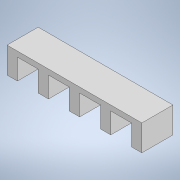
# Autodesk Inventor part: chamber
Saved by Autodesk Inventor 2021 (Build 250183000, 183)
## iProperties
Created: 2022-01-02
Part Number: chamber
Material: 一般
Document SubType Name: Modeling
Designer: shibu
Density: 1 g/cm^3
Appearance: 既定
Author: shibu
Autodesk Inventor part; units mm, degrees
ref_plane "YZ Plane" through (0, 0, 0) normal (1, 0, 0) x (0, 1, 0)
ref_plane "XZ Plane" through (0, 0, 0) normal (0, 1, 0) x (-1, 0, 0)
ref_plane "XY Plane" through (0, 0, 0) normal (0, 0, 1) x (1, 0, 0)
sketch "スケッチ1" plane through (0, 0, 0) normal (0, 0, 1) x (1, 0, 0)
  line L0 (0, 0) -> (-15, 0)
  line L1 (-15, 0) -> (-15, 20)
  line L2 (-15, 20) -> (0, 20)
  line L3 (0, 20) -> (0, 0)
  line L4 (0, 0) -> (0, 43.6966) construction
  line L5 (-15, 12.5) -> (-20, 12.5)
  line L6 (-20, 12.5) -> (-20, 0)
  line L7 (-30, 0) -> (-30, 12.5)
  line L8 (-30, 0) -> (-20, 0)
  line L9 (23.8812, 0) -> (-169.724, 0) construction
  line L10 (-45, 0) -> (-45, 12.5)
  line L11 (-45, 0) -> (-35, 0)
  line L12 (-35, 12.5) -> (-35, 0)
  line L13 (-30, 12.5) -> (-35, 12.5)
  line L14 (-60, 0) -> (-60, 12.5)
  line L15 (-60, 0) -> (-50, 0)
  line L16 (-50, 12.5) -> (-50, 0)
  line L17 (-45, 12.5) -> (-50, 12.5)
  line L18 (-75, 0) -> (-75, 12.5)
  line L19 (-75, 0) -> (-65, 0)
  line L20 (-65, 12.5) -> (-65, 0)
  line L21 (-60, 12.5) -> (-65, 12.5)
  line L22 (-75, 0) -> (-80, 0)
  line L23 (-80, 0) -> (-80, 20)
  line L24 (-80, 20) -> (-75, 20)
  line L25 (-75, 20) -> (-75, 0)
  line L26 (-75, 20) -> (-15, 20)
  line L27 (-75, 0) -> (-80, 5)
  line L28 (-75, 0) -> (-67.9289, 0) construction
  line L29 (0, 5) -> (-5, 0)
  line L30 (-40, 30.9864) -> (-40, -18.8288) construction
  line L31 (-42.5, 17.5) -> (-37.5, 17.5)
  line L32 (-37.5, 17.5) -> (-37.5, 5)
  line L33 (-37.5, 5) -> (-42.5, 5)
  line L34 (-42.5, 5) -> (-42.5, 17.5)
  line L35 (-42.5, 17.5) -> (-37.5, 5) construction
  line L36 (-37.5, 17.5) -> (-42.5, 5) construction
  line L37 (-57.5, 5) -> (-57.5, 17.5)
  line L38 (-52.5, 17.5) -> (-52.5, 5)
  line L39 (-52.5, 5) -> (-57.5, 5)
  line L40 (-72.5, 5) -> (-72.5, 17.5)
  line L41 (-67.5, 17.5) -> (-67.5, 5)
  line L42 (-67.5, 5) -> (-72.5, 5)
  line L43 (-27.5, 5) -> (-27.5, 17.5)
  line L44 (-22.5, 17.5) -> (-22.5, 5)
  line L45 (-22.5, 5) -> (-27.5, 5)
  line L46 (-42.5, 5) -> (-42.5, 17.5)
  line L47 (-37.5, 17.5) -> (-37.5, 5)
  line L48 (-37.5, 5) -> (-42.5, 5)
  line L49 (-57.5, 5) -> (-57.5, 17.5)
  line L50 (-52.5, 17.5) -> (-52.5, 5)
  line L51 (-52.5, 5) -> (-57.5, 5)
  line L52 (-12.5, 5) -> (-12.5, 17.5)
  line L53 (-7.5, 17.5) -> (-7.5, 5)
  line L54 (-7.5, 5) -> (-12.5, 5)
  line L55 (-27.5, 5) -> (-27.5, 17.5)
  line L56 (-22.5, 17.5) -> (-22.5, 5)
  line L57 (-22.5, 5) -> (-27.5, 5)
  line L58 (-42.5, 5) -> (-42.5, 17.5)
  line L59 (-37.5, 17.5) -> (-37.5, 5)
  line L60 (-37.5, 5) -> (-42.5, 5)
  line L61 (-72.5, 17.5) -> (-7.5, 17.5)
  line L62 (-72.5, 15) -> (-7.5, 15)
  point P0 (-40, 11.25)
  point P1 (-67.5, 15)
  point P2 (-57.5, 15)
  point P3 (-52.5, 15)
  point P4 (-42.5, 15)
  point P5 (-37.5, 15)
  point P6 (-27.5, 15)
  point P7 (-22.5, 15)
  point P8 (-12.5, 15)
  dimension "d4" = 15
  dimension "d5" = 20
  dimension "d6" = 5
  dimension "d7" = 10
  dimension "d8" = 7.5
  dimension "d9" = 15
  dimension "d10" = 5
  dimension "d11" = 135
  dimension "d12" = 5
  dimension "d13" = 135
  dimension "d17" = 12.5
  dimension "d18" = 5
  dimension "d19" = 5
  dimension "d22" = 15
  dimension "d25" = 15
  dimension "d28" = 2.5
  constraints: 126 end point, 14 point on line, 8 horizontal, 7 parallel, 6 perpendicular, 5 collinear, 2 midpoint, 2 vertical, 1 equal length, 84 other
  measures "d4" distance of L26.end L2.end
  measures "d5" distance of L0.end L26.end
  measures "d6" distance of L5.start L5.end
  measures "d7" distance between parallel lines of L6 L7
  measures "d8" distance between parallel lines of L5 L2
  measures "d9" distance of L7.start L10.start
  measures "d10" distance of L24.start L24.end
  measures "d11" angle of L28 L27
  measures "d12" distance from line of L9 L29.start
  measures "d13" angle of L0 L29
  measures "d17" distance between parallel lines of L33 L31
  measures "d18" distance between parallel lines of L9 L33
  measures "d19" distance between parallel lines of L32 L34
  measures "d22" distance of L33.end L37.start
  measures "d25" distance of L33.end L43.start
  measures "d28" distance between parallel lines of L62 L61
extrude "押し出し1" add sketch "スケッチ1" along normal blind 7.5 contours L62 L44 L61 L1 | L1 L61 L52 L62 | L62 L43 L61 L44 | L44 L45 L43 L62 | L62 L53 L54 L52 | L52 L61 L53 L62 | L62 L32 L61 L43 | L62 L34 L31 L32 | L32 L33 L34 L62 | L62 L38 L61 L34 | L62 L37 L61 L38 | L38 L39 L37 L62 | L62 L41 L61 L37 | L62 L40 L61 L41 | L41 L42 L40 L62
mirror "ミラー1" about plane through (-40, 11.25, 0) normal (0, 0, -1) of "押し出し1"
